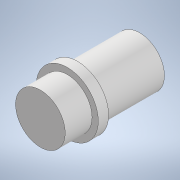
# Autodesk Inventor part: ClickHolder
Saved by Autodesk Inventor 2021 (Build 250183000, 183)
## iProperties
Created: 2021-07-10
Part Number: ClickHolder
Material: Generic
Document SubType Name: Modeling
Designer: teh18
Density: 1 g/cm^3
Appearance: Default
Author: teh18
Autodesk Inventor part; units mm, degrees
ref_plane "YZ Plane" through (0, 0, 0) normal (1, 0, 0) x (0, 1, 0)
ref_plane "XZ Plane" through (0, 0, 0) normal (0, 1, 0) x (-1, 0, 0)
ref_plane "XY Plane" through (0, 0, 0) normal (0, 0, 1) x (1, 0, 0)
sketch "Sketch1" plane through (0, 0, 0) normal (0, 0, 1) x (1, 0, 0)
  circle A0 centre (0, 0) radius 12
  dimension "d0" = 24
  constraints: 1 centre point, 1 coincident
  measures "d0" diameter of A0
extrude "Extrusion1" add sketch "Sketch1" along normal blind 30
sketch "Sketch2" plane through (0, 0, 30) normal (0, 0, 1) x (1, 0, 0)
  circle A0 centre (0, 0) radius 12 projected
  circle A1 centre (0, 0) radius 15
  dimension "d3" = 30
  constraints: 1 centre point, 1 coincident
  measures "d3" diameter of A1
extrude "Extrusion2" add sketch "Sketch2" along normal blind 5 contours A0 | A1
sketch "Sketch6" plane through (0, 0, 35) normal (0, 0, 1) x (1, 0, 0)
  circle A0 centre (0, 0) radius 3.75
  dimension "d20" = 7.5
  constraints: 1 centre point
  measures "d20" diameter of A0
extrude "Extrusion6" add sketch "Sketch6" along normal blind 18
ref_plane "Work Plane1" through (0, 0, 44) normal (0, 0, 1) x (1, 0, 0)
sketch "Sketch7" plane through (0, 0, 44) normal (0, 0, 1) x (1, 0, 0)
  line L0 (1.5, 3.75) -> (-1.5, 3.75)
  line L1 (-1.5, 3.75) -> (-1.5, -3.75)
  line L2 (-1.5, -3.75) -> (1.5, -3.75)
  line L3 (1.5, -3.75) -> (1.5, 3.75)
  line L4 (1.5, 3.75) -> (-1.5, -3.75) construction
  line L5 (-1.5, 3.75) -> (1.5, -3.75) construction
  point P0 (0, 0)
  dimension "d16" = 3
  dimension "d17" = 7.5
  constraints: 12 end point, 2 midpoint, 2 parallel, 1 horizontal, 1 perpendicular
  measures "d16" distance of L2.end L1.end
  measures "d17" distance of L1.end L0.end
extrude "Extrusion7" cut sketch "Sketch7" along normal blind 3
